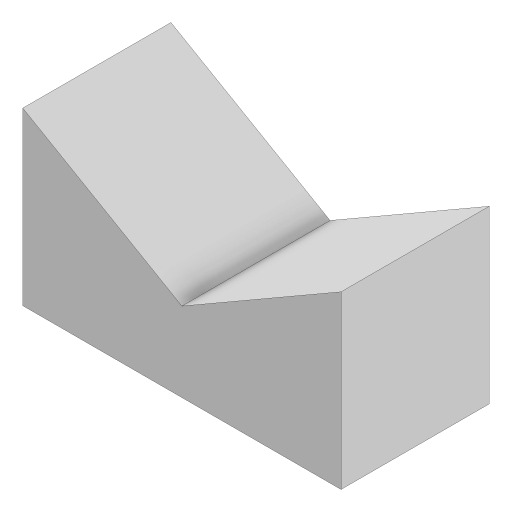
# Autodesk Inventor part: Cepek1
Saved by Autodesk Inventor 2023.3 (Build 273359000, 359)
## iProperties
Created: 2025-03-15
Part Number: Cepek1
Material: Generic
Document SubType Name: Modeling
Designer: David Zindović
Density: 1 g/cm^3
Appearance: Default
Author: David Zindović
Autodesk Inventor part; units mm, degrees
ref_plane "YZ Plane" through (0, 0, 0) normal (1, 0, 0) x (0, 1, 0)
ref_plane "XZ Plane" through (0, 0, 0) normal (0, 1, 0) x (-1, 0, 0)
ref_plane "XY Plane" through (0, 0, 0) normal (0, 0, 1) x (1, 0, 0)
sketch "Sketch1" plane through (0, 0, 0) normal (0, 0, 1) x (1, 0, 0)
  line L0 (0, 3.1754) -> (2.9, 1.5011)
  line L1 (2.75, 1.5877) -> (2.75, -1.5877)
  line L2 (2.9, -1.5011) -> (0, -3.1754)
  line L3 (0, -3.1754) -> (-2.9, -1.5011)
  line L4 (-2.75, -1.5877) -> (-2.75, 1.5877)
  line L5 (-2.9, 1.5011) -> (0, 3.1754)
  line L6 (-2.9, 3.1754) -> (2.9, 3.1754)
  line L7 (2.9, 3.1754) -> (2.9, -4.6199)
  line L8 (2.9, -4.6199) -> (-2.9, -4.6199)
  line L9 (-2.9, -4.6199) -> (-2.9, 3.1754)
  point P0 (0, 0)
  point P1 (0, 0)
  point P2 (0, 3.1754)
  dimension "d0" = 5.5
  dimension "d1" = 5.8
  dimension "d2" = 6.121
  constraints: 20 end point, 8 point on line, 3 coincident, 2 parallel, 1 horizontal, 1 midpoint, 1 perpendicular, 13 other
  measures "d0" distance between parallel lines of L1 L4
  measures "d1" distance between parallel lines of L9 L7
  measures "d2" distance of L5.start L8.end
extrude "Extrusion1" add sketch "Sketch1" along normal blind 2.7 contours L2 L7 L8 L9 L3
sketch "Sketch2" plane through (-2.9, -4.6199, 0) normal (0, -1, 0) x (1, 0, 0)
  line L0 (0.9, 2.3199) -> (1.9, 2.3199)
  line L1 (1.9, 2.3199) -> (1.9, 0.3199)
  line L2 (1.9, 0.3199) -> (0.9, 0.3199)
  line L3 (0.9, 0.3199) -> (0.9, 2.3199)
  line L4 (5.8, 0) -> (2.9, 0) projected
  line L5 (2.9, 0) -> (2.9, 0.3827)
  line L6 (2.9, 0) -> (2.9, 2.7) projected
  line L7 (4.9, 2.3199) -> (3.9, 2.3199)
  line L8 (3.9, 2.3199) -> (3.9, 0.3199)
  line L9 (3.9, 0.3199) -> (4.9, 0.3199)
  line L10 (4.9, 0.3199) -> (4.9, 2.3199)
  dimension "d5" = 1
  dimension "d6" = 1
  dimension "d7" = 2
  constraints: 18 end point, 4 symmetric about line, 2 parallel, 1 horizontal, 1 perpendicular, 1 point on line
  measures "d5" distance between parallel lines of L6 L1
  measures "d6" distance of L1.end L2.end
  measures "d7" distance of L0.end L1.end
extrude "Extrusion2" cut sketch "Sketch2" against normal blind 1.5
body "Solid1"
